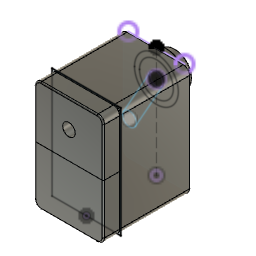
MUJI SHARPENER v0 (Autodesk Fusion 360 design; units mm, degrees)
Autodesk Fusion 360 part; units mm, degrees
sketch "Esquisse1" plane through (0, 0, 0) normal (0, 1, 0) x (1, 0, 0)
  line L0 (-27.5, 0) -> (27.5, 0)
  line L1 (27.5, 0) -> (27.5, -88.5)
  line L2 (27.5, -88.5) -> (-27.5, -88.5)
  line L3 (-27.5, -88.5) -> (-27.5, 0)
  dimension "d1" = 55
  dimension "d2" = 88.5
  constraint horizontal L0
  constraint vertical L1
  constraint horizontal L2
  constraint vertical L3
  constraint coincident L0 origin
  constraint midpoint L0 origin
  measures "d1" distance of L0.start L0.end
  measures "d2" distance of L0.end L1.end
extrude "Extrusion1" add sketch "Esquisse1" along normal blind 56 makes body 1
fillet "Congé1" radius 5 4 edges at (-27.5, 28, 88.5) (27.5, 28, 88.5) (-27.5, 28, 0) (27.5, 28, 0) on bodies 1
fillet "Congé2" radius 1 8 edges at (26.0355, 56, 87.0355) (27.5, 56, 44.25) (26.0355, 56, 1.4645) (0, 56, 0) (-26.0355, 56, 1.4645) (-27.5, 56, 44.25) (-26.0355, 56, 87.0355) (0, 56, 88.5) on bodies 1
shell "Coque1" thickness 2 removed faces 1 at (-9.1667, 0, 31.1667) on bodies 1
sketch "Esquisse2" plane through (0, 0, 0) normal (0, 1, 0) x (1, 0, 0)
  line L0 (-27.5, -45) -> (27.5, -45)
  line L1 (-27.5, 0) -> (27.5, 0)
  arc A0 (-27.5, -83.5) -> (-22.5, -88.5) centre (-22.5, -83.5) ccw
  line L2 (-27.5, -83.5) -> (-27.5, -5)
  arc A1 (-22.5, 0) -> (-27.5, -5) centre (-22.5, -5) ccw
  line L3 (-22.5, 0) -> (22.5, 0)
  arc A2 (27.5, -5) -> (22.5, 0) centre (22.5, -5) ccw
  line L4 (27.5, -5) -> (27.5, -83.5)
  line L5 (22.5, -88.5) -> (-22.5, -88.5)
  arc A3 (22.5, -88.5) -> (27.5, -83.5) centre (22.5, -83.5) ccw
  dimension "d10" = 45
  measures "d10" distance of L0 L1
extrude "Extrusion2" add sketch "Esquisse2" against normal blind 14 separate body contours L0 L1 L2 A1 L3 A2 L4 makes body 2
sketch "Esquisse3" plane through (0, 0, 0) normal (0, -1, 0) x (1, 0, 0)
  arc A0 (-25.5, 5) -> (-22.5, 2) centre (-22.5, 5) ccw
  line L0 (-25.5, 5) -> (-25.5, 83.5)
  arc A1 (-22.5, 86.5) -> (-25.5, 83.5) centre (-22.5, 83.5) ccw
  line L1 (-22.5, 86.5) -> (22.5, 86.5)
  arc A2 (25.5, 83.5) -> (22.5, 86.5) centre (22.5, 83.5) ccw
  line L2 (25.5, 83.5) -> (25.5, 5)
  arc A3 (22.5, 2) -> (25.5, 5) centre (22.5, 5) ccw
  line L3 (22.5, 2) -> (-22.5, 2)
  arc A4 (22.5, 0) -> (27.5, 5) centre (22.5, 5) ccw
  line L4 (27.5, 5) -> (27.5, 83.5)
  arc A5 (27.5, 83.5) -> (22.5, 88.5) centre (22.5, 83.5) ccw
  line L5 (22.5, 88.5) -> (-22.5, 88.5)
  arc A6 (-22.5, 88.5) -> (-27.5, 83.5) centre (-22.5, 83.5) ccw
  line L6 (-27.5, 83.5) -> (-27.5, 5)
  arc A7 (-27.5, 5) -> (-22.5, 0) centre (-22.5, 5) ccw
  line L7 (-22.5, 0) -> (22.5, 0)
  line L8 (-25.5, 5) -> (-25.5, 83.5)
  arc A8 (-25.5, 5) -> (-22.5, 2) centre (-22.5, 5) ccw
  line L9 (22.5, 2) -> (-22.5, 2)
  arc A9 (22.5, 2) -> (25.5, 5) centre (22.5, 5) ccw
  line L10 (25.5, 83.5) -> (25.5, 5)
  arc A10 (-22.5, 86.5) -> (-25.5, 83.5) centre (-22.5, 83.5) ccw
  line L11 (-22.5, 86.5) -> (22.5, 86.5)
  arc A11 (25.5, 83.5) -> (22.5, 86.5) centre (22.5, 83.5) ccw
  line L12 (-27.5, 45) -> (27.5, 45)
extrude "Extrusion3" add sketch "Esquisse3" against normal up to surface (54 mm away) contours A0 L0 L2 A3 L3 L8 A8 L9 A9 L10 L12 bodies 2
move_face "DécalerLesFaces1" offset -0.25 6 faces at (25.5, 36, 31.6667) (24, 36, 2.4019) (7.5, 18, 2) (-23.8747, 36, 2.3335) (-25.5, 36, 18.3333) (7.5, 54, 30.6667) on bodies 2
fillet "Congé3" radius 1 15 edges at (-27.5, -14, 25) (-26.0355, -14, 1.4645) (0, -14, 0) (26.0355, -14, 1.4645) (27.5, -14, 25) (-27.5, 0, 25) (-26.0355, 0, 1.4645) (0, 0, 0) (26.0355, 0, 1.4645) (27.5, 0, 25) (25.25, 53.75, 25) (24.4445, 53.75, 3.0555) (0, 53.75, 2.25) (-24.4445, 53.75, 3.0555) (-25.25, 53.75, 25) on bodies 2
fillet "Congé6" radius 0.5 5 edges at (-25.25, 0, 25) (-24.4445, 0, 3.0555) (0, 0, 2.25) (24.4445, 0, 3.0555) (25.25, 0, 25) on bodies 2
shell "Coque2" thickness 2 removed faces 1 at (-8.4167, 17.9167, 45) on bodies 2
extrude "Extrusion4" add sketch "Esquisse2" against normal up to surface (14 mm away) separate body contours L0 A0 L2 L4 L5 A3 makes body 3
extrude "Extrusion5" add sketch "Esquisse3" against normal up to surface (54 mm away) contours L0 A1 L1 A2 L2 L8 L10 A10 L11 A11 L12 bodies 3
move_face "DécalerLesFaces2" offset -0.25 6 faces at (25.5, 36, 70.6667) (24.6712, 36, 85.5702) (-7.5, 18, 86.5) (-24.3545, 36, 85.8582) (-25.5, 36, 57.8333) (7.5, 54, 58.8333) on bodies 3
fillet "Congé4" radius 1 10 edges at (27.5, 0, 64.25) (26.0355, 0, 87.0355) (0, 0, 88.5) (-26.0355, 0, 87.0355) (-27.5, 0, 64.25) (-27.5, -14, 64.25) (-26.0355, -14, 87.0355) (0, -14, 88.5) (26.0355, -14, 87.0355) (27.5, -14, 64.25) on bodies 3
fillet "Congé5" radius 0.5 5 edges at (25.25, 0, 64.25) (24.4445, 0, 85.4445) (0, 0, 86.25) (-24.4445, 0, 85.4445) (-25.25, 0, 64.25) on bodies 3
sketch "Esquisse5" plane through (0, -14, 0) normal (0, -1, 0) x (1, 0, 0)
  line L0 (26.5, 45) -> (26.5, 83.5)
  arc A0 (26.5, 83.5) -> (22.5, 87.5) centre (22.5, 83.5) ccw
  line L1 (22.5, 87.5) -> (-22.5, 87.5)
  arc A1 (-22.5, 87.5) -> (-26.5, 83.5) centre (-22.5, 83.5) ccw
  line L2 (-26.5, 83.5) -> (-26.5, 45)
  line L3 (-26.5, 45) -> (26.5, 45)
  circle A2 centre (0, 66.75) radius 5
  line L4 (0, 66.75) -> (0, 45)
  line L5 (0, 66.75) -> (0, 88.5)
  line L6 (22.5, 88.5) -> (-22.5, 88.5)
  dimension "d30" = 10
  constraint coincident A2.centre L4.start
  constraint midpoint L3 L4.end
  constraint perpendicular L3 L4
  constraint coincident L5.end L6
  constraint midpoint L5.end L6
  constraint equal L4 L5
  measures "d30" diameter of A2
extrude "Extrusion6" cut sketch "Esquisse5" against normal through all contours A2 L4 L5 | A2 L4 L5 bodies 3
shell "Coque3" thickness 2 removed faces 2 at (8.4167, 18.25, 45) at (-18.4814, 53.75, 64.8349) on bodies 3
move_face "DécalerLesFaces3" offset -5 1 faces at (6.2887, 53.75, 66.1538) on bodies 3
sketch "Esquisse6" plane through (0, 56, 0) normal (0, 1, 0) x (-1, 0, 0)
  arc A0 (-22.5, 87.5) -> (-26.5, 83.5) centre (-22.5, 83.5) ccw
  line L0 (-26.5, 83.5) -> (-26.5, 5)
  arc A1 (-26.5, 5) -> (-22.5, 1) centre (-22.5, 5) ccw
  line L1 (-22.5, 1) -> (22.5, 1)
  arc A2 (22.5, 1) -> (26.5, 5) centre (22.5, 5) ccw
  line L2 (26.5, 5) -> (26.5, 83.5)
  arc A3 (26.5, 83.5) -> (22.5, 87.5) centre (22.5, 83.5) ccw
  line L3 (22.5, 87.5) -> (-22.5, 87.5)
  circle A4 centre (0, 66.75) radius 17.5
  circle A5 centre (0, 66.75) radius 13.5
  circle A6 centre (0, 66.75) radius 5.5
  line L4 (-4.7925, 64.0514) -> (16.796, 25.7117)
  line L5 (4.7925, 69.4486) -> (26.3809, 31.1088)
  circle A7 centre (21.5884, 28.4102) radius 5.5
  line L6 (0, 88.5) -> (0, 0) construction
  line L7 (-22.5, 88.5) -> (22.5, 88.5)
  circle A8 centre (0, 66.75) radius 5
  dimension "d34" = 35
  dimension "d35" = 27
  dimension "d36" = 11
  dimension "d37" = 44
  constraint concentric A4 A5
  constraint concentric A5 A6
  constraint coincident A6 L4.start
  constraint coincident A6 L5.start
  constraint parallel L4 L5
  constraint tangent A6 L5
  constraint tangent A6 L4
  constraint coincident L5.end A7
  constraint coincident L4.end A7
  constraint tangent L4 A7
  constraint tangent L5 A7
  constraint coincident L6.end origin
  constraint perpendicular L1 L6
  constraint coincident L6.start L7
  constraint coincident A4.centre L6
  constraint concentric A6 A8
  measures "d34" diameter of A4
  measures "d35" diameter of A5
  measures "d36" diameter of A6
  measures "d37" distance of A4.centre A7.centre
extrude "Extrusion7" add sketch "Esquisse6" along normal blind 8 separate body contours A4 A5 L4 L5 | A4 A5 L4 L5 | A5 A6 L4 L5 | A5 A6 L4 L5 | A6 | A8 makes body 4
extrude "Extrusion8" add sketch "Esquisse6" along normal blind 7 from surface at 8 separate body contours A5 A6 L4 L5 | A5 A6 L4 L5 | A6 | A8 makes body 5
extrude "Extrusion9" add sketch "Esquisse6" along normal blind 4 from surface at 9.5 contours L2 A7 | L2 A7 | A4 L4 L5 A7 | A4 A5 L4 L5 | A5 A6 L4 L5 | A6 | A8 picked at (7.9204, 52.6838) picked at (8.1845, 59.6866) bodies 5
extrude "Extrusion10" add sketch "Esquisse6" along normal blind 11 from surface at 13.5 separate body contours L2 A7 | L2 A7 makes body 6
fillet "Congé7" radius 0.5 11 edges at (16.3157, 64, 60.4217) (16.3157, 56, 60.4217) (12.5864, 71, 61.8682) (-9.0263, 69.5, 39.5101) (-24.287, 69.5, 23.6177) (-18.6112, 69.5, 44.9072) (-9.0263, 65.5, 39.5101) (-24.287, 65.5, 23.6177) (-18.6112, 65.5, 44.9072) (-16.4606, 80.5, 26.4213) (-16.4606, 69.5, 30.3991) on bodies 4 5 6
equation "d37 = 49.5 mm - ( 11 / 2 ) * 1 mm"
equation "d43 = ( -( 7 - 4 ) / 2 ) * 1 mm"
named bodies: "MAIN BODY", "SHAVINGS", "SHARPENER", "HANDLE SUPPORT", "HANDLE", "HANDLE END"
